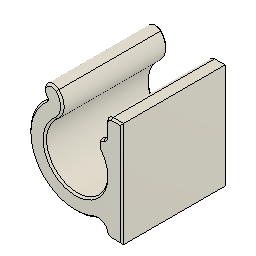
Hose holder D7 v3 (Autodesk Fusion 360 design; units mm, degrees)
Autodesk Fusion 360 part; units mm, degrees
note: some values were not read from the file. Chosen so that the rebuilt part matches the saved one: which pieces of a blend or face edit are solid. Set by a fixed rule: which sketch regions a step uses.
sketch "Náčrt1" plane through (0, 0, 0) normal (0, 0, 1) x (1, 0, 0)
  circle A0 centre (0, 0) radius 3.5
  circle A1 centre (0, 0) radius 5.3
  line L0 (3.5, 6) -> (3.5, -6)
  line L1 (5.3, 6) -> (5.3, -6)
  line L2 (3.5, 6) -> (5.3, 6)
  line L3 (3.5, -6) -> (5.3, -6)
  line L4 (-1.5, 6) -> (-1.5, 0) construction
  circle A2 centre (-3.5, 4.2426) radius 2
  circle A3 centre (-3.5, 4.2426) radius 0.2
  line L5 (-3.5, 4.2426) -> (-2.0858, 5.6569) construction
  line L6 (-3.5, 4.2426) -> (-1.5, 4.2426) construction
  circle A4 centre (-2.7222, 5.0205) radius 0.9
  circle A5 centre (3.5, 2.6665) radius 0.9
  point P0 (3.5, 0)
  dimension "d1" = 7
  dimension "d2" = 10.6
  dimension "d3" = 12
  dimension "d4" = 5
  dimension "d5" = 4
  dimension "d6" = 45
  constraint coincident A0.centre A1.centre
  constraint concentric A0 A1
  constraint vertical L0
  constraint midpoint L0 P0
  constraint horizontal A0.centre P0
  constraint tangent A0 L0
  constraint vertical L1
  constraint equal L0 L1
  constraint perpendicular L0 L2
  constraint tangent A1 L1
  constraint vertical L4
  constraint tangent A0 A2
  constraint tangent L4 A2
  constraint horizontal L0.start L4.start
  constraint horizontal A0.centre L4.end
  constraint concentric A2 A3
  constraint tangent A1 A3
  constraint horizontal L6
  constraint coincident A2.centre A3.centre
  constraint coincident L5 A4.centre
  constraint tangent A2 A4
  constraint tangent A3 A4
  constraint vertical L4.end L6.end
  constraint coincident L0 A5.centre
  constraint tangent A1 A5
  constraint tangent A0 A5
  measures "d1" diameter of A0
  measures "d2" diameter of A1
  measures "d3" distance of L0.start L0.end
  measures "d4" distance of L0 L4
  measures "d5" diameter of A2
  measures "d6" angle of L5 L6
extrude "Vysunutí1" add sketch "Náčrt1" along normal blind 12 contours A0 A1 L0 A2 | A0 L0 A5 | A1 L0 A5 | L0 A5 | A1 A2 A4 | L0 A5 | A1 L0 L1 L3 | A1 L0 A5 | A1 L0 L1 L2 | A1 A3 A4 | A1 A2 A4 | A1 A4 | A1 A4
fillet "Zaoblení1" radius 0.6 2 edges at (3.5, -6, 6) (3.5, 6, 6)
fillet "Zaoblení1" radius 1 1 edges at (3.5, -3.9799, 6)
fillet "Zaoblení1" radius 0.4 1 edges at (3.5, 3.5665, 6)
chamfer "Zkosení2" distance 0.2 angle 45 2 faces at (4.6974, 0.0779, 0) (4.6974, 0.0779, 12)
named bodies: "HoseHolderD7"
